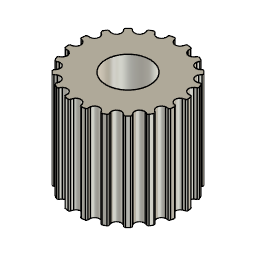
PC_v2 (Autodesk Fusion 360 design; units mm, degrees)
part number: 2026-03-17-17-27-52-163
Autodesk Fusion 360 part; units mm, degrees
note: some values were not read from the file. Set by a fixed rule: which sketch regions a step uses.
sketch "Sketch3" plane through (0, 0, 0) normal (0, 0, 1) x (1, 0, 0)
  circle A0 centre (0, 0) radius 6.1122
  line L0 (0, 6.1122) -> (0, 5.9172)
  circle A1 centre (0, 5.9172) radius 0.555
  line L1 (0, 6.1122) -> (-0.4, 6.1122)
  line L2 (0, 6.1122) -> (0.4, 6.1122)
  circle A2 centre (0, 6.1122) radius 0.6028
  line L3 (-0.7499, 6.066) -> (-5.5713, 5.5295)
  line L4 (0.7499, 6.066) -> (5.5713, 5.5295)
  arc A3 (0.7499, 6.066) -> (0.5855, 5.9424) centre (0.7333, 5.9169) ccw
  arc A4 (-0.5855, 5.9424) -> (-0.7499, 6.066) centre (-0.7333, 5.9169) ccw
  arc A5 (0.4989, 5.674) -> (-1.3872, 5.9527) centre (-0.4, 6.1122) ccw
  arc A6 (1.3872, 5.9527) -> (-0.4989, 5.674) centre (0.4, 6.1122) ccw
  circle A7 centre (-1.8285, 5.6276) radius 0.555
  arc A8 (-1.2789, 5.5505) -> (-3.1588, 5.2327) centre (-2.2692, 5.6894) ccw
  arc A9 (-1.1613, 6.0009) -> (-1.2795, 5.8325) centre (-1.131, 5.8539) ccw
  arc A10 (-0.5202, 6.09) -> (-2.2278, 5.2421) centre (-1.5084, 5.9367) ccw
  arc A11 (-2.3931, 5.4706) -> (-2.5877, 5.5374) centre (-2.5258, 5.4007) ccw
  circle A12 centre (-3.478, 4.7871) radius 0.555
  arc A13 (-2.9315, 4.8836) -> (-4.6212, 4.0005) centre (-3.9163, 4.7098) ccw
  arc A14 (-2.9588, 5.3483) -> (-3.0192, 5.1516) centre (-2.8846, 5.2179) ccw
  arc A15 (-2.3766, 5.6312) -> (-3.7387, 4.2971) centre (-3.2691, 5.18) ccw
  arc A16 (-3.9665, 4.4634) -> (-4.1722, 4.4667) centre (-4.0711, 4.3559) ccw
  circle A17 centre (-4.7871, 3.478) radius 0.555
  arc A18 (-4.2971, 3.7387) -> (-5.6312, 2.3766) centre (-5.18, 3.2691) ccw
  arc A19 (-4.4667, 4.1722) -> (-4.4634, 3.9665) centre (-4.3559, 4.0711) ccw
  arc A20 (-4.0005, 4.6212) -> (-4.8836, 2.9315) centre (-4.7098, 3.9163) ccw
  arc A21 (-5.1516, 3.0192) -> (-5.3483, 2.9588) centre (-5.2179, 2.8846) ccw
  circle A22 centre (-5.6276, 1.8285) radius 0.555
  arc A23 (-5.2421, 2.2278) -> (-6.09, 0.5202) centre (-5.9367, 1.5084) ccw
  arc A24 (-5.5374, 2.5877) -> (-5.4706, 2.3931) centre (-5.4007, 2.5258) ccw
  arc A25 (-5.2327, 3.1588) -> (-5.5505, 1.2789) centre (-5.6894, 2.2692) ccw
  arc A26 (-5.8325, 1.2795) -> (-6.0009, 1.1613) centre (-5.8539, 1.131) ccw
  circle A27 centre (-5.9172, 0) radius 0.555
  arc A28 (-5.674, 0.4989) -> (-5.9527, -1.3872) centre (-6.1122, -0.4) ccw
  arc A29 (-6.066, 0.7499) -> (-5.9424, 0.5855) centre (-5.9169, 0.7333) ccw
  arc A30 (-5.9527, 1.3872) -> (-5.674, -0.4989) centre (-6.1122, 0.4) ccw
  arc A31 (-5.9424, -0.5855) -> (-6.066, -0.7499) centre (-5.9169, -0.7333) ccw
  circle A32 centre (-5.6276, -1.8285) radius 0.555
  arc A33 (-5.5505, -1.2789) -> (-5.2327, -3.1588) centre (-5.6894, -2.2692) ccw
  arc A34 (-6.0009, -1.1613) -> (-5.8325, -1.2795) centre (-5.8539, -1.131) ccw
  arc A35 (-6.09, -0.5202) -> (-5.2421, -2.2278) centre (-5.9367, -1.5084) ccw
  arc A36 (-5.4706, -2.3931) -> (-5.5374, -2.5877) centre (-5.4007, -2.5258) ccw
  circle A37 centre (-4.7871, -3.478) radius 0.555
  arc A38 (-4.8836, -2.9315) -> (-4.0005, -4.6212) centre (-4.7098, -3.9163) ccw
  arc A39 (-5.3483, -2.9588) -> (-5.1516, -3.0192) centre (-5.2179, -2.8846) ccw
  arc A40 (-5.6312, -2.3766) -> (-4.2971, -3.7387) centre (-5.18, -3.2691) ccw
  arc A41 (-4.4634, -3.9665) -> (-4.4667, -4.1722) centre (-4.3559, -4.0711) ccw
  circle A42 centre (-3.478, -4.7871) radius 0.555
  arc A43 (-3.7387, -4.2971) -> (-2.3766, -5.6312) centre (-3.2691, -5.18) ccw
  arc A44 (-4.1722, -4.4667) -> (-3.9665, -4.4634) centre (-4.0711, -4.3559) ccw
  arc A45 (-4.6212, -4.0005) -> (-2.9315, -4.8836) centre (-3.9163, -4.7098) ccw
  arc A46 (-3.0192, -5.1516) -> (-2.9588, -5.3483) centre (-2.8846, -5.2179) ccw
  circle A47 centre (-1.8285, -5.6276) radius 0.555
  arc A48 (-2.2278, -5.2421) -> (-0.5202, -6.09) centre (-1.5084, -5.9367) ccw
  arc A49 (-2.5877, -5.5374) -> (-2.3931, -5.4706) centre (-2.5258, -5.4007) ccw
  arc A50 (-3.1588, -5.2327) -> (-1.2789, -5.5505) centre (-2.2692, -5.6894) ccw
  arc A51 (-1.2795, -5.8325) -> (-1.1613, -6.0009) centre (-1.131, -5.8539) ccw
  circle A52 centre (0, -5.9172) radius 0.555
  arc A53 (-0.4989, -5.674) -> (1.3872, -5.9527) centre (0.4, -6.1122) ccw
  arc A54 (-0.7499, -6.066) -> (-0.5855, -5.9424) centre (-0.7333, -5.9169) ccw
  arc A55 (-1.3872, -5.9527) -> (0.4989, -5.674) centre (-0.4, -6.1122) ccw
  arc A56 (0.5855, -5.9424) -> (0.7499, -6.066) centre (0.7333, -5.9169) ccw
  circle A57 centre (1.8285, -5.6276) radius 0.555
  arc A58 (1.2789, -5.5505) -> (3.1588, -5.2327) centre (2.2692, -5.6894) ccw
  arc A59 (1.1613, -6.0009) -> (1.2795, -5.8325) centre (1.131, -5.8539) ccw
  arc A60 (0.5202, -6.09) -> (2.2278, -5.2421) centre (1.5084, -5.9367) ccw
  arc A61 (2.3931, -5.4706) -> (2.5877, -5.5374) centre (2.5258, -5.4007) ccw
  circle A62 centre (3.478, -4.7871) radius 0.555
  arc A63 (2.9315, -4.8836) -> (4.6212, -4.0005) centre (3.9163, -4.7098) ccw
  arc A64 (2.9588, -5.3483) -> (3.0192, -5.1516) centre (2.8846, -5.2179) ccw
  arc A65 (2.3766, -5.6312) -> (3.7387, -4.2971) centre (3.2691, -5.18) ccw
  arc A66 (3.9665, -4.4634) -> (4.1722, -4.4667) centre (4.0711, -4.3559) ccw
  circle A67 centre (4.7871, -3.478) radius 0.555
  arc A68 (4.2971, -3.7387) -> (5.6312, -2.3766) centre (5.18, -3.2691) ccw
  arc A69 (4.4667, -4.1722) -> (4.4634, -3.9665) centre (4.3559, -4.0711) ccw
  arc A70 (4.0005, -4.6212) -> (4.8836, -2.9315) centre (4.7098, -3.9163) ccw
  arc A71 (5.1516, -3.0192) -> (5.3483, -2.9588) centre (5.2179, -2.8846) ccw
  circle A72 centre (5.6276, -1.8285) radius 0.555
  arc A73 (5.2421, -2.2278) -> (6.09, -0.5202) centre (5.9367, -1.5084) ccw
  arc A74 (5.5374, -2.5877) -> (5.4706, -2.3931) centre (5.4007, -2.5258) ccw
  arc A75 (5.2327, -3.1588) -> (5.5505, -1.2789) centre (5.6894, -2.2692) ccw
  arc A76 (5.8325, -1.2795) -> (6.0009, -1.1613) centre (5.8539, -1.131) ccw
  circle A77 centre (5.9172, 0) radius 0.555
  arc A78 (5.674, -0.4989) -> (5.9527, 1.3872) centre (6.1122, 0.4) ccw
  arc A79 (6.066, -0.7499) -> (5.9424, -0.5855) centre (5.9169, -0.7333) ccw
  arc A80 (5.9527, -1.3872) -> (5.674, 0.4989) centre (6.1122, -0.4) ccw
  arc A81 (5.9424, 0.5855) -> (6.066, 0.7499) centre (5.9169, 0.7333) ccw
  circle A82 centre (5.6276, 1.8285) radius 0.555
  arc A83 (5.5505, 1.2789) -> (5.2327, 3.1588) centre (5.6894, 2.2692) ccw
  arc A84 (6.0009, 1.1613) -> (5.8325, 1.2795) centre (5.8539, 1.131) ccw
  arc A85 (6.09, 0.5202) -> (5.2421, 2.2278) centre (5.9367, 1.5084) ccw
  arc A86 (5.4706, 2.3931) -> (5.5374, 2.5877) centre (5.4007, 2.5258) ccw
  circle A87 centre (4.7871, 3.478) radius 0.555
  arc A88 (4.8836, 2.9315) -> (4.0005, 4.6212) centre (4.7098, 3.9163) ccw
  arc A89 (5.3483, 2.9588) -> (5.1516, 3.0192) centre (5.2179, 2.8846) ccw
  arc A90 (5.6312, 2.3766) -> (4.2971, 3.7387) centre (5.18, 3.2691) ccw
  arc A91 (4.4634, 3.9665) -> (4.4667, 4.1722) centre (4.3559, 4.0711) ccw
  circle A92 centre (3.478, 4.7871) radius 0.555
  arc A93 (3.7387, 4.2971) -> (2.3766, 5.6312) centre (3.2691, 5.18) ccw
  arc A94 (4.1722, 4.4667) -> (3.9665, 4.4634) centre (4.0711, 4.3559) ccw
  arc A95 (4.6212, 4.0005) -> (2.9315, 4.8836) centre (3.9163, 4.7098) ccw
  arc A96 (3.0192, 5.1516) -> (2.9588, 5.3483) centre (2.8846, 5.2179) ccw
  circle A97 centre (1.8285, 5.6276) radius 0.555
  arc A98 (2.2278, 5.2421) -> (0.5202, 6.09) centre (1.5084, 5.9367) ccw
  arc A99 (2.5877, 5.5374) -> (2.3931, 5.4706) centre (2.5258, 5.4007) ccw
  arc A100 (3.1588, 5.2327) -> (1.2789, 5.5505) centre (2.2692, 5.6894) ccw
  arc A101 (1.2795, 5.8325) -> (1.1613, 6.0009) centre (1.131, 5.8539) ccw
  circle A102 centre (0, 0) radius 2.5
  line L5 (0, 0) -> (0, 5.9172)
  line L6 (0, 0) -> (2.5, 0)
  point P0 (0.602, 6.0825)
  point P1 (-0.602, 6.0825)
  dimension "d79" = 12.2244
  dimension "d80" = 0.195
  dimension "d81" = 1.11
  dimension "d82" = 0.4
  dimension "d83" = 0.4
  dimension "d84" = 2
  dimension "d85" = 2
  dimension "d86" = 1.2055
  dimension "d87" = 5
  dimension "d88" = 5
  dimension "d89" = 0.15
  dimension "d90" = 0.15
  dimension "d92" = 360
  dimension "d95" = 5
  constraint coincident A0.centre A102.centre
  constraint coincident A0 L0.start
  constraint vertical L0
  constraint coincident L0.end A1.centre
  constraint perpendicular L0 L1
  constraint perpendicular L0 L2
  constraint coincident L1.end A5.centre
  constraint coincident L2.end A6.centre
  constraint coincident A0 P0
  constraint coincident L0.start L1.start
  constraint coincident P0 A2
  constraint coincident A2 P1
  constraint coincident A0 P1
  constraint coincident P0 L4
  constraint tangent L4 A3
  constraint coincident A3.end A5
  constraint coincident A0 L4.start
  constraint coincident P1 L3
  constraint tangent L3 A4
  constraint coincident A4.start A6
  constraint coincident A0 L3.start
  constraint coincident A0 A5.end
  constraint coincident A1 A6.end
  constraint coincident A1 A5.start
  constraint coincident A0 A6.start
  constraint concentric A0 A102
  constraint tangent A3 A5
  constraint tangent A4 A6
  constraint parallel L0 L5
  constraint coincident A102 L6.end
  constraint perpendicular L5 L6
  measures "d79" diameter of A0
  measures "d80" distance of L0.start L0.end
  measures "d81" diameter of A1
  measures "d82" distance of L0.start L1.end
  measures "d83" distance of L0.start L2.end
  measures "d84" diameter of A5
  measures "d85" diameter of A6
  measures "d86" diameter of A2
  measures "d87" distance of P1 L3.end
  measures "d88" distance of P0 L4.end
  measures "d89" radius of A3
  measures "d90" radius of A4
  measures "d95" diameter of A102
extrude "Extrude6" add sketch "Sketch3" along normal blind 11 contours A0 A1 A3 A4 A5 A6 A7 A8 A9 A10 A11 A12 A13 A14 A15 A16 A17 A18 A19 A20 A21 A22 A23 A24 A25 A26 A27 A28 A29 A30 A31 A32 A33 A34 A35 A36 A37 A38 A39 A40 A41 A42 A43 A44 A45 A46 A47 A48 A49 A50 A51 A52 A53 A54 A55 A56 A57 A58 A59 A60 A61 A62 A63 A64 A65 A66 A67 A68 A69 A70 A71 A72 A73 A74 A75 A76 A77 A78 A79 A80 A81 A82 A83 A84 A85 A86 A87 A88 A89 A90 A91 A92 A93 A94 A95 A96 A97 A98 A99 A100 A101
equation "teeth = 20" comment "Enter # of teeth on pulley Note: When changing the # of teeth, if teeth are missing edit the extrude, remove all selections, then select the correct area."
equation "bore = 5 mm" comment "Enter bore diameter"
equation "pw = if(beltwidth == 9 mm; 11 mm; if(beltwidth == 10 mm; 11 mm; beltwidth + 1 mm))"
equation "beltwidth = 9 mm" comment "Enter belt width"
equation "pb = if(bore >= ( pd - 2 mm ); 5 mm; bore)"
equation "bt = if(teeth < 16; 16; teeth)"
equation "BeltPitch = 2" comment "2GT and 3GT supported"
equation "PLD = ( if(BeltPitch == 2; 0.254; 0.381) ) * 1 mm"
equation "pd = ( ( bt * BeltPitch / ( PI ) ) * 1 mm ) - ( PLD * 2 )"
equation "RootRadius = ( if(BeltPitch == 2; 0.555; 0.85) ) * 1 mm"
equation "FlankRadius = ( if(BeltPitch == 2; 1; 1.52) ) * 1 mm"
equation "ToothRadius = ( if(BeltPitch == 2; 0.15; 0.25) ) * 1 mm"
equation "FlankOffset = ( if(BeltPitch == 2; 0.4; 0.61) ) * 1 mm"
equation "ToothHeight = ( if(BeltPitch == 2; 0.75; 1.14) ) * 1 mm"
equation "d79 = pd"
equation "d80 = ToothHeight - RootRadius"
equation "d81 = RootRadius * 2"
equation "d82 = FlankOffset"
equation "d83 = FlankOffset"
equation "d84 = FlankRadius * 2"
equation "d85 = FlankRadius * 2"
equation "d89 = ToothRadius"
equation "d90 = ToothRadius"
equation "d91 = teeth"
equation "d93 = pw"
equation "d95 = bore"
